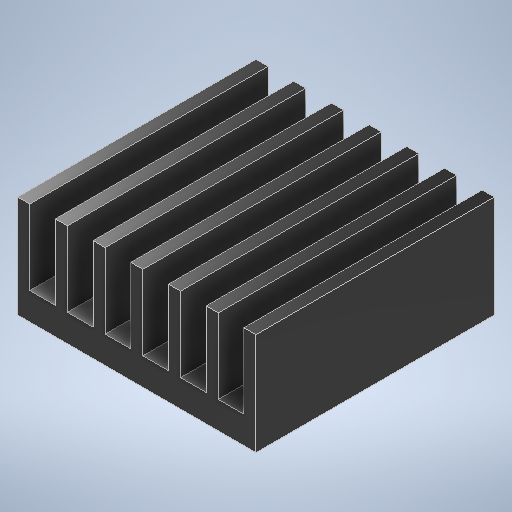
# Autodesk Inventor part: HEATSINK14x14
Saved by Autodesk Inventor 2025 (Build 290162000, 162)
## iProperties
Created: 2025-03-09
Part Number: HEATSINK14x14
Material: Aluminum 6061
Document SubType Name: Modeling
Designer: tvoko
Density: 2.7 g/cm^3
Appearance: Glossy - Black
Author: tvoko
Autodesk Inventor part; units mm, degrees
ref_plane "YZ Plane" through (0, 0, 0) normal (1, 0, 0) x (0, 1, 0)
ref_plane "XZ Plane" through (0, 0, 0) normal (0, 1, 0) x (-1, 0, 0)
ref_plane "XY Plane" through (0, 0, 0) normal (0, 0, 1) x (1, 0, 0)
sketch "Sketch1" plane through (0, 0, 0) normal (0, 1, 0) x (-1, 0, 0)
  line L0 (0, 0) -> (-14, 0)
  line L1 (-14, 0) -> (-14, -14)
  line L2 (-14, -14) -> (0, -14)
  line L3 (0, -14) -> (0, 0)
  dimension "d0" = 14
  dimension "d1" = 14
  constraints: 8 end point, 2 parallel, 1 horizontal, 1 perpendicular
  measures "d0" distance of L2.end L1.end
  measures "d1" distance of L1.end L0.end
extrude "Extrusion1" add sketch "Sketch1" along normal blind 6
sketch "Sketch2" plane through (0, 0, 0) normal (0, 0, 1) x (1, 0, 0)
  line L0 (0, 0) -> (14, 0) projected
  line L1 (14, 0) -> (14, 6) projected
  line L2 (0, 6) -> (14, 6) projected
  line L3 (0, 0) -> (0, 6) projected
  line L4 (0.7143, 6) -> (2.2143, 6)
  line L5 (2.2143, 6) -> (2.2143, 1.6)
  line L6 (2.2143, 1.6) -> (0.7143, 1.6)
  line L7 (0.7143, 1.6) -> (0.7143, 6)
  line L8 (0.7143, 3.8) -> (0, 3.8) construction
  line L9 (4.4286, 6) -> (4.4286, 1.6)
  line L10 (4.4286, 1.6) -> (2.9286, 1.6)
  line L11 (2.9286, 1.6) -> (2.9286, 6)
  line L12 (2.9286, 3.8) -> (2.2143, 3.8) construction
  line L13 (6.6429, 6) -> (6.6429, 1.6)
  line L14 (6.6429, 1.6) -> (5.1429, 1.6)
  line L15 (5.1429, 1.6) -> (5.1429, 6)
  line L16 (5.1429, 3.8) -> (4.4286, 3.8) construction
  line L17 (8.8571, 6) -> (8.8571, 1.6)
  line L18 (8.8571, 1.6) -> (7.3571, 1.6)
  line L19 (7.3571, 1.6) -> (7.3571, 6)
  line L20 (7.3571, 3.8) -> (6.6429, 3.8) construction
  line L21 (11.0714, 6) -> (11.0714, 1.6)
  line L22 (11.0714, 1.6) -> (9.5714, 1.6)
  line L23 (9.5714, 1.6) -> (9.5714, 6)
  line L24 (9.5714, 3.8) -> (8.8571, 3.8) construction
  line L25 (0, 6) -> (14, 6) projected
  line L26 (13.2857, 6) -> (13.2857, 1.6)
  line L27 (13.2857, 1.6) -> (11.7857, 1.6)
  line L28 (11.7857, 1.6) -> (11.7857, 6)
  line L29 (11.7857, 3.8) -> (11.0714, 3.8) construction
  line L30 (13.2857, 3.8) -> (14, 3.8) construction
  dimension "d4" = 6
  dimension "d5" = 1.6
  dimension "d6" = 1.5
  dimension "d8" = 1.5
  dimension "d9" = 1.5
  dimension "d10" = 1.5
  dimension "d11" = 1.5
  dimension "d12" = 1.5
  constraints: 52 end point, 17 perpendicular, 12 midpoint, 11 equal length, 7 parallel, 7 point on line, 1 horizontal, 7 other
  measures "d4" distance of L0.start L2.start
  measures "d5" distance between parallel lines of L0 L6
  measures "d6" distance between parallel lines of L7 L5
  measures "d8" distance between parallel lines of L11 L9
  measures "d9" distance between parallel lines of L15 L13
  measures "d10" distance between parallel lines of L19 L17
  measures "d11" distance between parallel lines of L23 L21
  measures "d12" distance between parallel lines of L28 L26
extrude "Extrusion2" cut sketch "Sketch2" against normal through all contours L2 L5 L6 L7 | L26 L27 L28 L2 | L2 L9 L10 L11 | L21 L22 L23 L2 | L2 L13 L14 L15 | L17 L18 L19 L2
body "Solid1"
